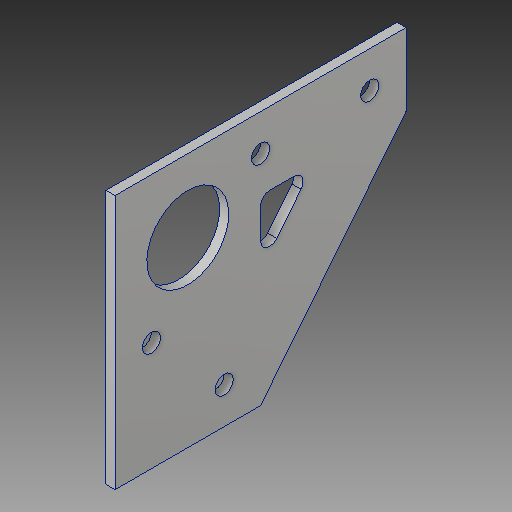
# Autodesk Inventor part: 15102898-16-P-0205_CPY
Saved by Autodesk Inventor 2017 (Build 210142000, 142)
## iProperties
Created: 2016-10-02
Part Number: 15102898-16-P-0205_CPY
Material: Aluminum 6061
Document SubType Name: Modeling
Designer: gus
Mass: 55.4711 g
Surface Area: 147.521 cm^2
Volume: 20.5448 cm^3
Density: 2.7 g/cm^3
Appearance: Aluminum - Flat
Author: gus
Autodesk Inventor part; units mm, degrees
ref_plane "YZ Plane" through (0, 0, 0) normal (1, 0, 0) x (0, 1, 0)
ref_plane "XZ Plane" through (0, 0, 0) normal (0, 1, 0) x (-1, 0, 0)
ref_plane "XY Plane" through (0, 0, 0) normal (0, 0, 1) x (1, 0, 0)
sketch "Sketch1" plane through (0, 0, 0) normal (1, 0, 0) x (0, 1, 0)
  line L0 (0, 0) -> (0, -101.6)
  line L1 (0, -101.6) -> (-25.4, -101.6)
  line L2 (-25.4, -101.6) -> (-88.9, -50.8)
  line L3 (-88.9, -50.8) -> (-88.9, 0)
  circle A0 centre (-50.8, -12.7) radius 3.175
  circle A1 centre (-12.7, -50.8) radius 3.175
  circle A2 centre (-12.7, -88.9) radius 3.175
  line L4 (-12.7, -25.4) -> (-12.7, -101.6) construction
  line L5 (0, -12.7) -> (-88.9, -12.7) construction
  circle A3 centre (-76.2, -38.1) radius 3.175
  circle A4 centre (-25.4, -25.4) radius 14.2875
  line L6 (0, 0) -> (-88.9, 0)
  dimension "d0" = 50.8
  dimension "d1" = 25.4
  dimension "d2" = 88.9
  dimension "d3" = 101.6
  dimension "d5" = 38.1
  dimension "d6" = 12.7
  dimension "d10" = 12.7
  dimension "d11" = 12.7
  dimension "d13" = 28.575
  dimension "d15" = 6.35
  dimension "d24" = 90
  dimension "d25" = 12.7
  dimension "d26" = 25.4
  dimension "d27" = 76.2
  dimension "d29" = 63.5
  dimension "d30" = 6.35
  dimension "d31" = 50.8
  dimension "d32" = 38.1
  constraints: 14 end point, 5 centre point, 5 point on line, 3 perpendicular, 2 equal radius, 1 midpoint, 1 parallel, 1 vertical
  measures "d0" distance of L3.end L2.end
  measures "d1" distance of L0.end L1.end
  measures "d2" distance of L3.end L0.start
  measures "d3" distance of L0.start L0.end
  measures "d5" distance of A2.centre A1.centre
  measures "d6" distance between parallel lines of L0 L4
  measures "d10" distance from line of L3 A3.centre
  measures "d11" horizontal distance of A3.centre L2.end
  measures "d13" diameter of A4
  measures "d15" diameter of A1
  measures "d24" angle of L0 L6
  measures "d25" distance between parallel lines of L6 L5
  measures "d26" distance from line of A4.centre L6
  measures "d27" distance from line of L4.start L1
  measures "d29" distance from line of L3 A4.centre
  measures "d30" diameter of A0
  measures "d31" distance from line of L0 A0.centre
  measures "d32" distance from line of A1.centre L5
extrude "Extrusion1" add sketch "Sketch1" along normal blind 3.175
sketch "Sketch2" plane through (3.175, 0, 0) normal (1, 0, 0) x (0, 0, -1)
  line L0 (50.8, -39.1889) -> (50.8, -28.575)
  line L1 (53.975, -25.4) -> (62.4661, -25.4)
  line L2 (64.9454, -30.5584) -> (56.4543, -41.1723)
  line L3 (101.6, 0) -> (0, 0) projected
  line L4 (0, 0) -> (0, -101.6) projected
  line L5 (50.8, -88.9) -> (101.6, -25.4) projected
  arc A0 (50.8, -39.1889) -> (56.4543, -41.1723) centre (53.975, -39.1889) ccw
  arc A1 (53.975, -25.4) -> (50.8, -28.575) centre (53.975, -28.575) ccw
  arc A2 (64.9454, -30.5584) -> (62.4661, -25.4) centre (62.4661, -28.575) ccw
  line L6 (0, 0) -> (0, -88.9) projected
  dimension "d18" = 25.4
  dimension "d19" = 25.4
  dimension "d21" = 3.175
  dimension "d28" = 50.8
  constraints: 6 end point, 6 point on circle, 6 tangent, 3 centre point, 3 parallel, 2 equal radius
  measures "d18" distance between parallel lines of L2 L5
  measures "d19" distance between parallel lines of L3 L1
  measures "d21" radius of A0
  measures "d28" distance between parallel lines of L6 L0
extrude "Extrusion2" cut sketch "Sketch2" against normal blind 3.175
body "Solid1"
